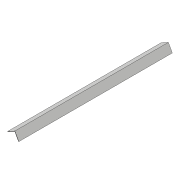
# Autodesk Inventor part: Barra freno
Saved by Autodesk Inventor 2020 (Build 240168000, 168)
## iProperties
Created: 2020-02-07
Part Number: Barra freno
Material: Generic
Document SubType Name: Modeling
Designer: Juan Carlos Botero
Density: 1 g/cm^3
Appearance: Default
Mass: 331.935 g
Surface Area: 2686.19 cm^2
Volume: 331.935 cm^3
Author: Juan Carlos Botero
Autodesk Inventor part; units mm, degrees
ref_plane "YZ Plane" through (0, 0, 0) normal (1, 0, 0) x (0, 1, 0)
ref_plane "XZ Plane" through (0, 0, 0) normal (0, 1, 0) x (-1, 0, 0)
ref_plane "XY Plane" through (0, 0, 0) normal (0, 0, 1) x (1, 0, 0)
sketch "Sketch1" plane through (0, 0, 0) normal (0, 0, 1) x (1, 0, 0)
  circle A0 centre (-76.4616, -331.0553) radius 285.0725 projected
  line L0 (42.2033, -71.8546) -> (14.6776, -21.3711)
  line L1 (14.6776, -21.3711) -> (-35.8059, -48.8968)
  line L2 (-35.8059, -48.8968) -> (-37.0027, -46.7018)
  line L3 (-37.0027, -46.7018) -> (15.6758, -17.9794)
  line L4 (15.6758, -17.9794) -> (44.3982, -70.6579)
  line L5 (44.3982, -70.6579) -> (42.2033, -71.8546)
  dimension "d15" = 2.5
  dimension "d16" = 60
  constraints: 12 end point, 6 perpendicular, 2 point on circle, 1 parallel
  measures "d15" distance of L4.end L0.start
  measures "d16" distance of L3.end L4.end
extrude "Extrusion1" add sketch "Sketch1" along normal mid plane 1120 contours L0 L1 L2 L3 L4 L5
sketch "Sketch3" plane through (0, 0, 0) normal (0, 0, 1) x (1, 0, 0)
  circle A0 centre (2.6996, -62.0716) radius 5
  circle A1 centre (2.6996, -62.0716) radius 10
  line L0 (-35.8059, -48.8968) -> (14.6776, -21.3711) projected
  line L1 (14.6776, -21.3711) -> (42.2033, -71.8546) projected
  line L2 (7.4867, -70.8513) -> (33.8259, -56.4901)
  line L3 (33.8259, -56.4901) -> (18.4879, -28.3595)
  line L4 (18.4879, -28.3595) -> (7.6892, -25.1814)
  line L5 (7.6892, -25.1814) -> (-20.4414, -40.5194)
  line L6 (-20.4414, -40.5194) -> (-6.0802, -66.8586)
  point P0 (0, 0)
  dimension "d21" = 10
  dimension "d22" = 20
  dimension "d25" = 40
  constraints: 10 end point, 4 perpendicular, 3 point on line, 2 centre point, 2 point on circle, 2 tangent, 1 coincident, 1 parallel
  measures "d21" diameter of A0
  measures "d22" diameter of A1
  measures "d25" distance between parallel lines of L1 L6
extrude "Extrusion4" add sketch "Sketch3" along normal mid plane 6 separate body contours A1 | A1 L6 L0 L4 L1 L2
